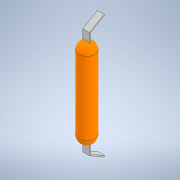
# Autodesk Inventor part: LED Filament
Saved by Autodesk Inventor 2022 (Build 260153000, 153)
## iProperties
Created: 2022-01-31
Part Number: LED Filament
Material: Generic
Document SubType Name: Modeling
Designer: tecware
Density: 1 g/cm^3
Appearance: Default
Author: tecware
Autodesk Inventor part; units mm, degrees
ref_plane "YZ Plane" through (0, 0, 0) normal (1, 0, 0) x (0, 1, 0)
ref_plane "XZ Plane" through (0, 0, 0) normal (0, 1, 0) x (-1, 0, 0)
ref_plane "XY Plane" through (0, 0, 0) normal (0, 0, 1) x (1, 0, 0)
sketch "Sketch1" plane through (0, 0, 0) normal (0, 0, 1) x (1, 0, 0)
  line L0 (1, 4.5) -> (1, -4.5)
  line L1 (-1, -4.5) -> (-1, 4.5)
  arc A0 (1, 4.5) -> (-1, 4.5) centre (0, 4.5) ccw
  arc A1 (-1, -4.5) -> (1, -4.5) centre (0, -4.5) ccw
  line L2 (0, 5.5) -> (0, -5.5)
  point P0 (0, 0)
  point P1 (0, 0)
  dimension "d0" = 2
  dimension "d1" = 9
  constraints: 6 end point, 6 point on circle, 2 centre point, 1 midpoint, 1 parallel
  measures "d0" distance of L0.end L1.start
  measures "d1" distance of L0.start L0.end
revolve "Revolution1" add sketch "Sketch1" angle 360 about axis through (0, 5.5, 0) along (0, -1, 0) contours L2 A1 L1 A0
sketch "Sketch3" plane through (0, 0, 0) normal (1, 0, 0) x (0, 1, 0)
  line L0 (8.5, 0.075) -> (4.5, 0.075)
  line L1 (4.5, 0.075) -> (4.5, -0.075)
  line L2 (4.5, -0.075) -> (8.5, -0.075)
  line L3 (8.5, -0.075) -> (8.5, 0.075)
  line L4 (0, 1.5086) -> (0, -1.8047) construction
  line L5 (6.5, -0.075) -> (7.5, -1.8071)
  line L6 (6.5, -0.075) -> (8.5, -0.075) construction
  line L7 (7.5, -1.8071) -> (7.6299, -1.7321)
  line L8 (7.6299, -1.7321) -> (6.5866, 0.075)
  line L9 (-8.5, 0.075) -> (-4.5, 0.075)
  line L10 (-4.5, 0.075) -> (-4.5, -0.075)
  line L11 (-4.5, -0.075) -> (-8.5, -0.075)
  line L12 (-8.5, -0.075) -> (-8.5, 0.075)
  line L13 (-6.5, -0.075) -> (-7.5, -1.8071)
  line L14 (-6.5, -0.075) -> (-8.5, -0.075) construction
  line L15 (-7.5, -1.8071) -> (-7.6299, -1.7321)
  line L16 (-7.6299, -1.7321) -> (-6.5866, 0.075)
  point P0 (0, 0)
  dimension "d7" = 4
  dimension "d8" = 0.15
  dimension "d11" = 2
  dimension "d12" = 60
  dimension "d13" = 0.15
  dimension "d14" = 4.5
  constraints: 34 end point, 10 symmetric about line, 6 point on line, 3 horizontal, 3 perpendicular, 2 parallel, 2 vertical, 1 equal length, 1 midpoint
  measures "d7" distance of L2.end L1.end
  measures "d8" distance of L1.end L0.end
  measures "d11" distance of L5.start L5.end
  measures "d12" angle of L5 L6
  measures "d13" distance of L5.end L7.end
  measures "d14" distance from line of L4 L1.end
extrude "Extrusion2" add sketch "Sketch3" along normal mid plane 0.8 contours L8 L2 L1 L0 | L8 L7 L5 L2 | L9 L10 L11 L16 | L11 L13 L15 L16
body "Solid1"
